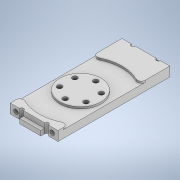
# Autodesk Inventor part: Leg_joint_basis_frame
Saved by Autodesk Inventor 2020.4 (Build 244396000, 396)
## iProperties
Created: 2021-09-21
Part Number: Leg_joint_basis_frame
Material: 一般
Document SubType Name: Modeling
Designer: Masato
Density: 1 g/cm^3
Appearance: 滑らか - 淡い灰色
Author: Masato
Autodesk Inventor part; units mm, degrees
ref_plane "YZ Plane" through (0, 0, 0) normal (1, 0, 0) x (0, 1, 0)
ref_plane "XZ Plane" through (0, 0, 0) normal (0, 1, 0) x (-1, 0, 0)
ref_plane "XY Plane" through (0, 0, 0) normal (0, 0, 1) x (1, 0, 0)
sketch "スケッチ1" plane through (0, 0, 0) normal (0, 0, 1) x (1, 0, 0)
  line L0 (-12.5, 29.25) -> (12.5, 29.25)
  line L1 (12.5, 29.25) -> (12.5, -29.25)
  line L2 (12.5, -29.25) -> (-12.5, -29.25)
  line L3 (-12.5, -29.25) -> (-12.5, 29.25)
  line L4 (-12.5, 29.25) -> (12.5, -29.25) construction
  line L5 (12.5, 29.25) -> (-12.5, -29.25) construction
  line L6 (-5.5, 29.25) -> (-5.5, 31.25)
  line L7 (-5.5, 31.25) -> (5.5, 31.25)
  line L8 (0, 29.25) -> (0, -29.25) construction
  line L9 (5.5, 29.25) -> (5.5, 31.25)
  arc A0 (-7.6, 29.25) -> (-5.5, 29.25) centre (-6.55, 29.25) ccw
  arc A1 (5.5, 29.25) -> (7.6, 29.25) centre (6.55, 29.25) ccw
  line L10 (-12.5, 0) -> (12.5, 0) construction
  line L11 (-5.5, -29.25) -> (-5.5, -31.25)
  line L12 (-5.5, -31.25) -> (5.5, -31.25)
  line L13 (5.5, -29.25) -> (5.5, -31.25)
  arc A2 (-5.5, -29.25) -> (-7.6, -29.25) centre (-6.55, -29.25) ccw
  arc A3 (7.6, -29.25) -> (5.5, -29.25) centre (6.55, -29.25) ccw
  circle A4 centre (0, -5) radius 21.75
  circle A5 centre (0, 3) radius 1.3
  circle A6 centre (-6.9282, -1) radius 1.3
  circle A7 centre (-6.9282, -9) radius 1.3
  circle A8 centre (0, -13) radius 1.3
  circle A9 centre (6.9282, -9) radius 1.3
  circle A10 centre (6.9282, -1) radius 1.3
  circle A11 centre (0, -5) radius 10.75
  circle A12 centre (0, -5) radius 21.5 construction
  line L14 (-12.5, -26.75) -> (12.5, -26.75) construction
  point P0 (0, 0)
  point P1 (12.5, -22.7992)
  point P2 (-12.5, -22.7992)
  point P3 (-5.5, -29.25)
  point P4 (5.5, -29.25)
  point P5 (-12.5, 12.7992)
  point P6 (12.5, 12.7992)
  point P7 (7.6, 29.25)
  point P8 (5.5, -29.25)
  point P9 (-5.5, -29.25)
  dimension "d0" = 25
  dimension "d1" = 58.5
  dimension "d2" = 11
  dimension "d3" = 2
  dimension "d4" = 1.05
  dimension "d6" = 2.6
  dimension "d10" = 360
  dimension "d13" = 21.5
  dimension "d14" = 43
  dimension "d15" = 0.25
  dimension "d17" = 24.25
  dimension "d18" = 8
  dimension "d19" = 2.5
  constraints: 30 end point, 13 centre point, 12 symmetric about line, 8 point on circle, 7 point on line, 6 midpoint, 4 perpendicular, 2 coincident, 2 parallel, 1 horizontal, 1 tangent, 16 other
  measures "d0" distance of L1.end L2.end
  measures "d1" distance of L0.end L1.end
  measures "d2" distance of L7.end L6.end
  measures "d3" vertical distance of L0.end L7.end
  measures "d4" radius of A0
  measures "d6" diameter of A5
  measures "d13" diameter of A11
  measures "d14" diameter of A12
  measures "d15" radial gap between concentric circles of A12 A4
  measures "d17" distance of L8.end A11.centre
  measures "d18" distance of A11.centre A5.centre
  measures "d19" distance of L2.end L14.start
extrude "押し出し1" add sketch "スケッチ1" along normal blind 5 contours L0 A0 A1 L1 A4 L3 | A4 L1 L2 A3 A2 L3 | A11
extrude "押し出し2" add sketch "スケッチ1" along normal blind 4 contours A4 L1 L3
extrude "押し出し3" add sketch "スケッチ1" along normal blind 2.5 contours L6 L7 L9 L0 | L2 L13 L12 L11
sketch "スケッチ2" plane through (-12.5, -29.25, 0) normal (0, -1, 0) x (1, 0, 0)
  line L0 (0, 0) -> (4.9, 0) projected
  line L1 (23.25, 5) -> (1.75, 5) projected
  line L2 (12.5, 5) -> (12.5, 0) construction
  point P0 (3, 2.5)
  point P1 (22, 2.5)
  dimension "d26" = 2.5
  dimension "d27" = 19
  constraints: 2 end point, 1 midpoint, 1 symmetric about line, 1 vertical
  measures "d26" distance from line of L0 point (3, 2.5)
  measures "d27" distance of point (22, 2.5) point (3, 2.5)
hole "穴1" at (-9.5, -29.25, 2.5) at (9.5, -29.25, 2.5) direction (0, 1, 0) diameter 2.459 depth 8 tip angle 118 thread size "M3x0.5" class "6H" standard "ISO Metric profile"
sketch "スケッチ3" plane through (-12.5, 29.25, 0) normal (0, 1, 0) x (1, 0, 0)
  circle A0 centre (22, -2.5) radius 1.2295 projected
  circle A1 centre (3, -2.5) radius 1.2295 projected
  point P0 (12.5, 0)
  constraints: 2 coincident
hole "穴2" at (9.5, 29.25, 2.5) at (-9.5, 29.25, 2.5) direction (0, -1, 0) diameter 2.459 depth 8 tip angle 118 thread size "M3x0.5" class "6H" standard "ISO Metric profile"
fillet "フィレット1" radius 2 4 edges at (-12.5, 12.7992, 4.5) (12.5, 12.7992, 4.5) (-12.5, -22.7992, 4.5) (12.5, -22.7992, 4.5)
